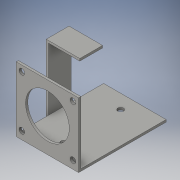
# Autodesk Inventor part: MotorClamp
Saved by Autodesk Inventor 2016 (Build 200138000, 138)
## iProperties
Created: 2016-11-29
Part Number: MotorClamp
Material: Generic
Document SubType Name: Sheet Metal
Designer: Evan Phil George
Density: 1 g/cm^3
Appearance: Light Gray
Sheet Metal Rule: Default
Author: Evan Phil George
Autodesk Inventor part; units mm, degrees
ref_plane "YZ Plane" through (0, 0, 0) normal (1, 0, 0) x (0, 1, 0)
ref_plane "XZ Plane" through (0, 0, 0) normal (0, 1, 0) x (-1, 0, 0)
ref_plane "XY Plane" through (0, 0, 0) normal (0, 0, 1) x (1, 0, 0)
sketch "Sketch1" plane through (0, 0, 0) normal (0, 0, 1) x (1, 0, 0)
  line L0 (-27.5, 27.5) -> (27.5, 27.5)
  line L1 (27.5, 27.5) -> (27.5, -27.5)
  line L2 (27.5, -27.5) -> (-27.5, -27.5)
  line L3 (-27.5, -27.5) -> (-27.5, 27.5)
  circle A0 centre (-22.5, 22.5) radius 2.5
  circle A1 centre (22.5, 22.5) radius 2.5
  circle A2 centre (-22.5, -22.5) radius 2.5
  circle A3 centre (22.5, -22.5) radius 2.5
  circle A4 centre (0, 0) radius 19.25
  dimension "d1" = 55
  dimension "d2" = 55
  dimension "d3" = 27.5
  dimension "d4" = 27.5
  dimension "d5" = 38.5
  dimension "d6" = 5
  dimension "d7" = 5
  dimension "d8" = 5
  dimension "d9" = 5
  dimension "d10" = 5
  dimension "d11" = 5
  dimension "d12" = 5
  dimension "d13" = 5
  dimension "d14" = 5
  dimension "d15" = 5
  dimension "d16" = 5
  dimension "d17" = 5
  constraints: 8 end point, 5 centre point, 2 parallel, 1 coincident, 1 horizontal, 1 perpendicular
  measures "d1" distance of L0.start L0.end
  measures "d2" distance of L0.end L1.end
  measures "d3" distance from line of point (0, 0) L1
  measures "d4" distance from line of point (0, 0) L0
  measures "d5" diameter of A4
  measures "d6" diameter of A0
  measures "d7" distance from line of A0.centre L0
  measures "d8" distance from line of L3 A0.centre
  measures "d9" diameter of A1
  measures "d10" distance from line of A1.centre L0
  measures "d11" distance from line of A1.centre L1
  measures "d12" diameter of A3
  measures "d13" distance from line of L2 A3.centre
  measures "d14" distance from line of A3.centre L1
  measures "d15" diameter of A2
  measures "d16" distance from line of L2 A2.centre
  measures "d17" distance from line of L3 A2.centre
extrude "Extrusion1" add sketch "Sketch1" along normal blind 2
sketch "Sketch2" plane through (27.5, -27.5, 0) normal (1, 0, 0) x (0, 0, -1)
  line L0 (0, 0) -> (-2, 0) projected
  line L1 (0, 0) -> (75, 0)
  line L2 (75, 0) -> (75, -2)
  line L3 (75, -2) -> (-2, -2)
  line L4 (-2, -2) -> (-2, 0)
  point P0 (0, 27.5)
  dimension "d20" = 75
  dimension "d21" = 2
  dimension "d22" = 77
  constraints: 8 end point, 2 horizontal, 1 vertical
  measures "d20" distance of L0.start L1.end
  measures "d21" distance of L1.end L2.end
  measures "d22" distance of L2.end L3.end
extrude "Extrusion2" add sketch "Sketch2" against normal blind 55
sketch "Sketch3" plane through (-27.5, -27.5, 0) normal (-1, 0, 0) x (0, 0, 1)
  line L0 (-75, -2) -> (2, -2) projected
  line L1 (-36.5, -2) -> (-36.5, 55)
  line L2 (0, 0) -> (-75, 0) projected
  line L3 (-36.5, 55) -> (-46.5, 55)
  line L4 (-46.5, 55) -> (-46.5, -2)
  line L5 (-46.5, -2) -> (-26.5, -2)
  line L6 (-26.5, -2) -> (-26.5, 55)
  line L7 (-26.5, 55) -> (-36.5, 55)
  point P0 (0, 27.5)
  dimension "d25" = 57
  dimension "d26" = 10
  dimension "d27" = 57
  dimension "d28" = 20
  dimension "d29" = 57
  constraints: 12 end point, 3 point on line, 1 collinear, 1 horizontal, 1 midpoint, 1 perpendicular
  measures "d25" distance of L1.start L1.end
  measures "d26" distance of L1.end L3.end
  measures "d27" distance of L3.end L4.end
  measures "d28" distance of L4.end L5.end
  measures "d29" distance of L5.end L6.end
extrude "Extrusion3" add sketch "Sketch3" along normal blind 2
sketch "Sketch4" plane through (-27.5, 27.5, -26.5) normal (0, 1, 0) x (1, 0, 0)
  line L0 (-2, 0) -> (-2, 20) projected
  line L1 (-2, 20) -> (27.5, 20)
  line L2 (27.5, 20) -> (27.5, 0)
  line L3 (0, 0) -> (-2, 0) projected
  line L4 (27.5, 0) -> (-2, 0)
  line L5 (-2, 0) -> (-2, 20)
  point P0 (27.5, -26.5)
  dimension "d32" = 29.5
  dimension "d33" = 20
  constraints: 8 end point, 1 collinear, 1 horizontal, 1 vertical
  measures "d32" distance of L0.end L1.end
  measures "d33" distance of L1.end L2.end
extrude "Extrusion4" add sketch "Sketch4" along normal blind 2
sketch "Sketch5" plane through (27.5, -27.5, 0) normal (0, 1, 0) x (1, 0, 0)
  line L0 (0, 75) -> (0, 0) projected
  line L1 (0, 37.5) -> (-27.5, 37.5)
  line L2 (-27.5, 37.5) -> (-27.5, 62.5)
  line L3 (-27.5, 26.5) -> (-27.5, 46.5) projected
  line L4 (-27.5, 37.5) -> (-27.5, 12.5)
  circle A0 centre (-27.5, 62.5) radius 2.5
  circle A1 centre (-27.5, 12.5) radius 2.5
  point P0 (-27.5, 0)
  dimension "d36" = 27.5
  dimension "d37" = 25
  dimension "d38" = 25
  dimension "d39" = 5
  dimension "d40" = 5
  constraints: 6 end point, 2 centre point, 2 coincident, 1 collinear, 1 horizontal, 1 midpoint, 1 point on line
  measures "d36" distance of L1.start L1.end
  measures "d37" distance of L1.end L2.end
  measures "d38" distance of L1.end L4.end
  measures "d39" diameter of A0
  measures "d40" diameter of A1
extrude "Extrusion5" cut sketch "Sketch5" against normal blind 2
equation "\"BendRadius\" = Thickness"
equation "\"BendReliefWidth\" = Thickness"
equation "\"BendReliefDepth\" = 0.5 * Thickness"
equation "\"CornerReliefSize\" = 4 * Thickness"
equation "\"MinimumRemnant\" = 2 * Thickness"
equation "\"TransitionRadius\" = BendRadius"
equation "\"JacobiRadiusSize\" = Thickness"
equation "\"GapSize\" = Thickness"
equation "\"Thickness\" = 0.5"
body "Solid1"
